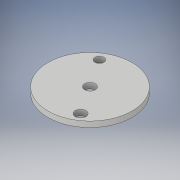
# Autodesk Inventor part: Giroservo
Saved by Autodesk Inventor 2019 (Build 230136000, 136)
## iProperties
Created: 2020-02-07
Part Number: Giroservo
Material: Generic
Document SubType Name: Modeling
Designer: Omar
Density: 1 g/cm^3
Appearance: Default
Author: Omar
Autodesk Inventor part; units mm, degrees
ref_plane "YZ Plane" through (0, 0, 0) normal (1, 0, 0) x (0, 1, 0)
ref_plane "XZ Plane" through (0, 0, 0) normal (0, 1, 0) x (-1, 0, 0)
ref_plane "XY Plane" through (0, 0, 0) normal (0, 0, 1) x (1, 0, 0)
sketch "Sketch1" plane through (0, 0, 0) normal (0, 1, 0) x (-1, 0, 0)
  circle A0 centre (0, 0) radius 15
  circle A1 centre (0, 0) radius 1.9
  circle A2 centre (6.6332, -10) radius 1.59
  circle A3 centre (-6.6332, 10) radius 1.9
  dimension "d0" = 30
  dimension "d1" = 3.8
  dimension "d2" = 3.18
  dimension "d3" = 12
  dimension "d4" = 10
  dimension "d10" = 12
  dimension "d11" = 3.8
  dimension "d12" = 10
  constraints: 4 centre point, 2 coincident
  measures "d0" diameter of A0
  measures "d1" diameter of A1
  measures "d2" diameter of A2
  measures "d3" distance of A2.centre A0.centre
  measures "d4" vertical distance of point (0, 0) A2.centre
  measures "d10" distance of point (0, 0) A3.centre
  measures "d11" diameter of A3
  measures "d12" vertical distance of point (0, 0) A3.centre
extrude "Extrusion1" add sketch "Sketch1" along normal blind 2
body "Solid1"
